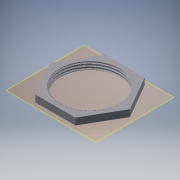
# Autodesk Inventor part: 27_Nut
Saved by Autodesk Inventor 2016 (Build 200138000, 138)
## iProperties
Created: 2016-12-20
Part Number: 27_Nut
Material: Generisch
Document SubType Name: Modeling
Designer: diederichbenedict
Density: 1 g/cm^3
Appearance: Vorgabe
Author: diederichbenedict
Autodesk Inventor part; units mm, degrees
ref_plane "YZ Plane" through (0, 0, 0) normal (1, 0, 0) x (0, 1, 0)
ref_plane "XZ Plane" through (0, 0, 0) normal (0, 1, 0) x (-1, 0, 0)
ref_plane "XY Plane" through (0, 0, 0) normal (0, 0, 1) x (1, 0, 0)
ref_plane "Arbeitsebene1" through (0, 0, 0) normal (0, 0, 1) x (1, 0, 0)
sketch "Skizze1" plane through (0, 0, 0) normal (0, 0, 1) x (1, 0, 0)
  line L0 (24.1976, -0.0885) -> (24.1976, 0.0885) construction
  line L1 (12.1244, 21) -> (24.1976, 0.0885) construction
  line L2 (-12.1244, 21) -> (12.1244, 21) construction
  line L3 (-24.2487, 0) -> (-12.1244, 21) construction
  line L4 (-12.1244, -21) -> (-24.2487, 0) construction
  line L5 (12.1244, -21) -> (-12.1244, -21) construction
  line L6 (24.1976, -0.0885) -> (12.1244, -21) construction
  circle A0 centre (0, 0) radius 18.5 construction
  line L7 (-11.8357, 20.5) -> (11.8357, 20.5)
  line L8 (11.8357, 20.5) -> (23.6714, 0)
  line L9 (23.6714, 0) -> (11.8357, -20.5)
  line L10 (11.8357, -20.5) -> (-11.8357, -20.5)
  line L11 (-11.8357, -20.5) -> (-23.6714, 0)
  line L12 (-23.6714, 0) -> (-11.8357, 20.5)
  circle A1 centre (0, 0) radius 18.75
  circle A2 centre (0, 0) radius 17.5 projected
  circle A3 centre (0, 0) radius 18
  point P0 (0, 0)
  dimension "d0" = 0.5
  dimension "d1" = 0.25
  dimension "d4" = 0.5
  constraints: 12 end point, 2 centre point, 5 other
  measures "d0" distance between parallel lines of L3 L12
  measures "d1" radial gap between concentric circles of A0 A1
  measures "d4" radial gap between concentric circles of A2 A3
extrude "Extrusion1" add sketch "Skizze1" along normal blind 4 contours L7 L8 L9 L10 L11 L12 | A1
thread "Gewinde1" size "M36x1.5" class "6H" standard "ANSI Metric M Profile" full length
sketch "Skizze3" plane through (0, 0, 4) normal (-1, 0, 0) x (0, 1, 0)
  line L0 (18, 0) -> (18, 4)
  line L1 (18, 4) -> (16.9874, 4)
  line L2 (16.9874, 4) -> (16.9874, 0)
  line L3 (16.9874, 0) -> (18, 0)
  line L4 (0, -0.8) -> (0, 4.8)
  line L5 (18, 4) -> (18, 0)
  spline S0 degree 3 number of poles 544 construction
  constraints: 8 end point, 1 point on line
revolve "Umdrehung1" add sketch "Skizze3" angle 360 about axis through (0, 0, 4) along (0, 0, -1) separate body
sketch "Skizze2" plane through (0, 17.25, 4) normal (1, 0, 0) x (0, 0, -1)
  line L0 (-1.2014, 0.5362) -> (-1.0627, 0.5362) construction
  line L1 (-0.1741, -0.2826) -> (-0.3127, -0.5227) construction
  line L2 (-1.8127, -0.5227) -> (-1.9514, -0.2826) construction
  line L3 (-0.9241, 0.5362) -> (-1.0627, 0.7763) construction
  line L4 (-1.0627, 0.7763) -> (-1.2014, 0.5362) construction
  line L5 (-1.8127, -0.5227) -> (-1.6741, -0.2826) construction
  line L6 (-0.9241, 0.5362) -> (-0.4514, -0.2826)
  line L7 (-1.9514, -0.2826) -> (-1.6741, -0.2826) construction
  arc A0 (-1.9514, -0.2826) -> (-1.8127, -0.3626) centre (-1.8127, -0.2025) ccw construction
  line L8 (-0.1741, -0.2826) -> (-0.4514, -0.2826) construction
  line L9 (-1.8127, -0.5227) -> (-1.8127, -0.2826) construction
  line L10 (-0.3127, -0.5227) -> (-0.3127, -0.2826) construction
  line L11 (-1.0627, 0.7763) -> (-1.0627, 0.6163) construction
  line L12 (-1.8127, -0.3626) -> (-0.3127, -0.3626)
  arc A1 (-1.8127, -0.3626) -> (-1.6741, -0.2826) centre (-1.8127, -0.2025) ccw
  line L13 (-0.4514, -0.2826) -> (-0.3127, -0.5227) construction
  line L14 (-1.6741, -0.2826) -> (-1.2014, 0.5362)
  line L15 (-0.3127, 0.6163) -> (-0.3127, 0.3871)
  line L16 (-0.3127, 0.3871) -> (-0.3127, 0.6163)
  line L17 (-0.3127, 0.6163) -> (-0.2793, 0.6163)
  arc A2 (-0.4514, -0.2826) -> (-0.3127, -0.3626) centre (-0.3127, -0.2025) ccw
  arc A3 (-0.3127, -0.3626) -> (-0.1741, -0.2826) centre (-0.3127, -0.2025) ccw construction
  arc A4 (-1.0627, 0.6163) -> (-1.2014, 0.5362) centre (-1.0627, 0.4562) ccw
  arc A5 (-0.9241, 0.5362) -> (-1.0627, 0.6163) centre (-1.0627, 0.4562) ccw
  line L18 (-1.0627, 0.6163) -> (-1.0627, 0.5362) construction
  line L19 (-1.0627, 0.5362) -> (-0.9241, 0.5362) construction
  line L20 (4, 0.75) -> (0, 0.75) projected
  line L21 (4, -0.2626) -> (0, -0.2626) projected
  dimension "d8" = 60
  dimension "d9" = 0.2401
  dimension "d10" = 0.2401
  dimension "Skizze2_ThreadOffset" = 0
  dimension "Skizze2_MajorRadius" = 0.9789
  dimension "d13" = 1.5
  dimension "Skizze2_MinorRadius" = 0
  dimension "d27" = 0.1
  constraints: 40 end point, 12 point on circle, 10 parallel, 8 tangent, 6 centre point, 6 collinear, 2 midpoint, 2 point on line, 1 horizontal, 1 perpendicular
  measures "d8" angle of L6 L14
  measures "d9" distance of L3.end L0.end
  measures "d10" distance of L1.end L10.end
  measures "Skizze2_ThreadOffset" distance between parallel lines of L15 L10
  measures "Skizze2_MajorRadius" distance from line of L12 L15.start
  measures "d13" distance from line of L1.end L9
  measures "Skizze2_MinorRadius" distance edge to line of A5 L17
  measures "d27" distance between parallel lines of L21 L12
coil "Spirale1" sketch "Skizze2" operation cut axis through (0, 0, 4) along (0, 0, -1) pitch 1.5015 turns 4.662005 hand right bodies 2
equation "\"d8\" = d15"
equation "\"d9\" = 0.160083 * Skizze2_Pitch"
equation "\"d10\" = 0.160083 * Skizze2_Pitch"
equation "\"d13\" = Skizze2_Pitch"
equation "\"d15\" = 60deg"
equation "\"Skizze2_Pitch\" = 1.5"
